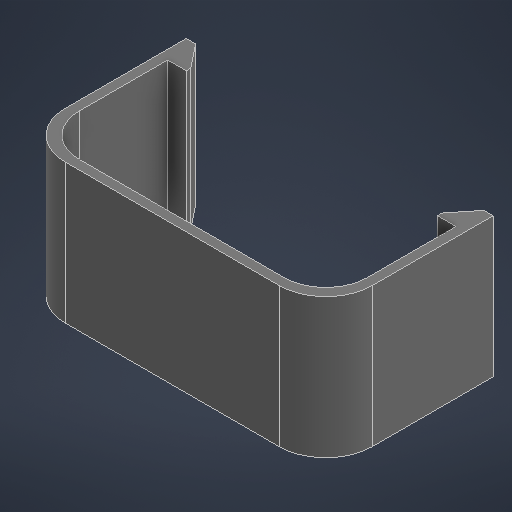
# Autodesk Inventor part: P_Halter
Saved by Autodesk Inventor 2026 (Build 300175000, 175)
## iProperties
Created: 2025-08-19
Part Number: P_Halter
Material: Generisch
Document SubType Name: Modeling
Designer: FAL
Density: 1 g/cm^3
Appearance: Vorgabe
Author: FAL
Autodesk Inventor part; units mm, degrees
ref_plane "YZ Plane" through (0, 0, 0) normal (1, 0, 0) x (0, 1, 0)
ref_plane "XZ Plane" through (0, 0, 0) normal (0, 1, 0) x (-1, 0, 0)
ref_plane "XY Plane" through (0, 0, 0) normal (0, 0, 1) x (1, 0, 0)
sketch "Skizze1" plane through (0, 0, 0) normal (0, 0, 1) x (1, 0, 0)
  line L0 (15.5, 18) -> (16.5, 18)
  line L1 (16.5, 18) -> (16.5, 5)
  line L2 (11.5, 0) -> (0, 0)
  line L3 (0, 0) -> (0, 1)
  line L4 (0, 1) -> (11, 1)
  line L5 (15.5, 5.5) -> (15.5, 15)
  line L6 (15.5, 15) -> (13.5, 15)
  line L7 (13.5, 15) -> (13.5, 15.5)
  line L8 (13.5, 15.5) -> (15.5, 18)
  arc A0 (11, 1) -> (15.5, 5.5) centre (11, 5.5) ccw
  arc A1 (11.5, 0) -> (16.5, 5) centre (11.5, 5) ccw
  point P0 (16.5, 0)
  point P1 (15.5, 1)
  point P2 (16, 18)
  dimension "d0" = 1
  dimension "d1" = 1
  dimension "d2" = 15.5
  dimension "d3" = 14
  dimension "d4" = 3
  dimension "d5" = 0.5
  dimension "d6" = 1
  dimension "d7" = 2
  dimension "d10" = 4.5
  dimension "d11" = 5
  constraints: 18 end point, 7 perpendicular, 4 point on circle, 4 point on line, 4 tangent, 2 centre point, 1 horizontal, 1 midpoint
  measures "d0" distance between parallel lines of L1 L5
  measures "d1" distance between parallel lines of L2 L4
  measures "d2" distance between parallel lines of L3 L5
  measures "d3" distance between parallel lines of L4 L6
  measures "d4" distance from line of point (16, 18) L6
  measures "d5" distance of L6.end L7.end
  measures "d6" distance of L0.start L0.end
  measures "d7" distance between parallel lines of L5 L7
  measures "d10" radius of A0
  measures "d11" radius of A1
extrude "Extrusion1" add sketch "Skizze1" along normal blind 15
mirror "Spiegeln1" about plane through (0, 0, 0) normal (1, 0, 0)
